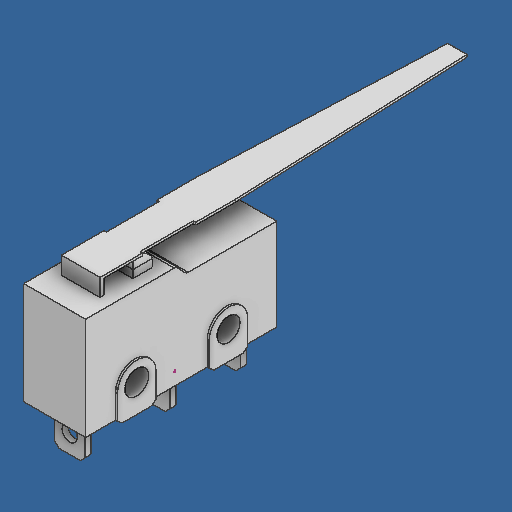
# Autodesk Inventor part: limit_switch
Saved by Autodesk Inventor 2026.2 (Build 302298000, 298)
## iProperties
Created: 2026-01-30
Part Number: limit_switch
Material: Generic
Document SubType Name: Modeling
Designer: Thoma
Density: 1 g/cm^3
Appearance: Default
Author: Thoma
Autodesk Inventor part; units mm, degrees
ref_plane "YZ Plane" through (0, 0, 0) normal (1, 0, 0) x (0, 1, 0)
ref_plane "XZ Plane" through (0, 0, 0) normal (0, 1, 0) x (-1, 0, 0)
ref_plane "XY Plane" through (0, 0, 0) normal (0, 0, 1) x (1, 0, 0)
sketch "Sketch4" plane through (0, 0, 0) normal (1, 0, 0) x (0, 1, 0)
  line L0 (9.275, 9.2) -> (-1.325, 9.2)
  line L1 (-1.325, 9.2) -> (-1.325, -10.6)
  line L2 (-1.325, -10.6) -> (9.275, -10.6)
  line L3 (9.275, -10.6) -> (9.275, 9.2)
  line L4 (-1.325, -0.7) -> (8.175, -0.7)
  line L5 (8.175, -0.7) -> (8.175, -10.6)
  line L6 (8.175, -10.6) -> (-1.325, -10.6)
  line L7 (-1.325, -10.6) -> (-1.325, -0.7)
  line L8 (9.275, -0.2) -> (8.175, -1.2)
  circle A0 centre (1.175, 4.1) radius 1.25
  line L9 (-1.725, 5.6) -> (-1.725, 2.6)
  line L10 (-1.725, 5.6) -> (-1.325, 6.1)
  line L11 (-1.725, 2.6) -> (-1.325, 2.1)
  line L12 (1.175, 4.1) -> (-1.325, 4.1)
  circle A1 centre (1.175, 4.1) radius 2
  line L13 (1.175, 6.1) -> (-1.325, 6.1)
  line L14 (1.175, 2.1) -> (-1.325, 2.1)
  circle A2 centre (1.175, -5.4) radius 1.2
  point P0 (0, 0)
  point P1 (9.275, -0.7)
  dimension "d11" = 10.6
  dimension "d12" = 9.5
  dimension "d13" = 0.5
  dimension "d14" = 0.5
  dimension "d15" = 19.8
  dimension "d16" = 2.5
  dimension "d17" = 2.5
  dimension "d18" = 5.1
  dimension "d19" = 0.4
  dimension "d20" = 2
  dimension "d21" = 2
  dimension "d22" = 0.5
  dimension "d23" = 0.5
  dimension "d24" = 4
  dimension "d37" = 9.5
  dimension "d38" = 2.4
  constraints: 30 end point, 6 point on line, 4 parallel, 3 centre point, 3 horizontal, 3 perpendicular, 2 coincident, 2 midpoint, 2 point on circle, 1 tangent, 1 vertical
  measures "d11" distance of L0.start L0.end
  measures "d12" distance of L4.start L4.end
  measures "d13" distance of L4.end L8.end
  measures "d14" distance of point (9.275, -0.7) L8.start
  measures "d15" distance of L0.end L1.end
  measures "d16" diameter of A0
  measures "d17" distance from line of L1 L12.start
  measures "d18" distance from line of L0 L12.start
  measures "d19" distance between parallel lines of L1 L9
  measures "d20" distance of L12.end L10.end
  measures "d21" distance of L11.end L12.end
  measures "d22" vertical distance of L10.end L9.start
  measures "d23" vertical distance of L11.end L9.end
  measures "d24" diameter of A1
  measures "d37" distance of point (1.175, -5.4) L12.start
  measures "d38" diameter of A2
extrude "Extrusion4" add sketch "Sketch4" against normal blind 6.4 contours L3 L8 L5 L4 L1 L14 A1 L13 L0 | L13 A1 L12 L1 | L1 L11 L9 L10 | L5 L2 L1 L4 | L12 A1 L14 L1 | A1
sketch "Sketch5" plane through (0, 0, 0) normal (1, 0, 0) x (0, 0, -1)
  line L0 (-6.1, -1.325) -> (-6.1, 1.102)
  line L1 (10.6, -1.325) -> (-2.1, -1.325) projected
  line L2 (-2.1, -1.325) -> (-2.1, 1.102)
  circle A0 centre (-4.1, 1.175) radius 1.25 projected
  arc A1 (-2.1, 1.175) -> (-6.1, 1.175) centre (-4.1, 1.175) ccw
  line L3 (-9.2, -1.325) -> (-6.1, -1.325) projected
  line L4 (-6.1, -1.325) -> (-5.6, -1.725) projected
  line L5 (-6.1, -1.325) -> (-5.6, -1.725)
  line L6 (-5.6, -1.725) -> (-2.6, -1.725) projected
  line L7 (-5.6, -1.725) -> (-2.6, -1.725)
  line L8 (-2.6, -1.725) -> (-2.1, -1.325)
  circle A2 centre (5.4, 1.175) radius 1.2
  arc A3 (7.4, 1.175) -> (3.4, 1.175) centre (5.4, 1.175) ccw
  line L9 (3.4, 1.175) -> (3.4, -1.325)
  line L10 (7.4, 1.175) -> (7.4, -1.325)
  line L11 (3.9, -1.725) -> (6.9, -1.725)
  line L12 (3.4, -1.325) -> (3.9, -1.725)
  line L13 (6.9, -1.725) -> (7.4, -1.325)
  line L14 (-6.1, 1.102) -> (-6.1, 1.175)
  line L15 (-2.1, 1.175) -> (-2.1, 1.102)
  point P0 (0, 0)
  dimension "d27" = 4
  dimension "d28" = 9.5
  dimension "d29" = 2.5
  dimension "d30" = 2.4
  dimension "d31" = 4
  dimension "d32" = 0.5
  dimension "d33" = 0.5
  dimension "d34" = 0.4
  constraints: 24 end point, 4 point on circle, 4 point on line, 4 vertical, 3 centre point, 3 coincident, 2 collinear, 2 perpendicular, 1 horizontal, 1 tangent
  measures "d27" diameter of A1
  measures "d28" distance of point (5.4, 1.175) A1.centre
  measures "d29" distance from line of L1 point (5.4, 1.175)
  measures "d30" diameter of A2
  measures "d31" diameter of A3
  measures "d32" horizontal distance of L9.end L11.start
  measures "d33" horizontal distance of L10.end L11.end
  measures "d34" distance between parallel lines of L11 L1
extrude "Extrusion5" add sketch "Sketch5" along normal blind 0.2
sketch "Sketch6" plane through (0, 0, 0) normal (1, 0, 0) x (0, 0, -1)
  point P0 (0, 0)
sketch "Sketch7" plane through (0, 0, 0) normal (-1, 0, 0) x (0, 0, 1)
  circle A0 centre (-5.4, 1.175) radius 1.2 projected
  line L0 (-3.9, -1.725) -> (-6.9, -1.725) projected
  line L1 (-5.4, 1.175) -> (-3.9, -1.725)
  line L2 (-3.4, -1.325) -> (-3.9, -1.725) projected
  line L3 (-3.9, -1.725) -> (-3.4, -1.325)
  line L4 (-7.4, -1.325) -> (-10.6, -1.325) projected
  line L5 (-3.4, -1.325) -> (-7.4, -1.325)
  line L6 (-7.4, -1.325) -> (-6.9, -1.725)
  line L7 (-6.9, -1.725) -> (-7.4, -1.325) projected
  point P0 (0, 0)
  constraints: 8 end point, 2 collinear, 1 point on line
extrude "Extrusion6" add sketch "Sketch7" along normal blind 6.4 contours L0 L6 L5 L1 | L1 L5 L2
fillet "Fillet1" radius 0.5 2 edges at (-3.2, 8.175, -1.2) (-3.2, 9.275, -0.2)
sketch "Sketch8" plane through (-6.4, 0, 0) normal (-1, 0, 0) x (0, 0, 1)
  circle A0 centre (-5.4, 1.175) radius 1.2 projected
  circle A1 centre (-5.4, 1.175) radius 1.2
  circle A2 centre (4.1, 1.175) radius 1.25 projected
  circle A3 centre (4.1, 1.175) radius 1.25
  circle A4 centre (-5.4, 1.175) radius 2
  circle A5 centre (4.1, 1.175) radius 2
  line L0 (-3.4, -1.325) -> (2.1, -1.325) projected
  line L1 (-3.4, -1.325) -> (-3.4, 1.175)
  line L2 (-10.6, -1.325) -> (-7.4, -1.325) projected
  line L3 (-7.4, 1.175) -> (-7.4, -1.325) projected
  line L4 (-7.4, -1.325) -> (-7.4, 1.175)
  line L5 (-7.4, -1.325) -> (-6.9, -1.725) projected
  line L6 (-7.4, -1.325) -> (-6.9, -1.725)
  line L7 (-6.9, -1.725) -> (-3.9, -1.725) projected
  line L8 (-6.9, -1.725) -> (-3.9, -1.725)
  line L9 (-3.9, -1.725) -> (-3.4, -1.325)
  line L10 (2.1, -1.325) -> (2.1, 1.175)
  line L11 (6.1, -1.325) -> (9.2, -1.325) projected
  line L12 (6.1, -1.325) -> (6.1, 1.175)
  line L13 (2.6, -1.725) -> (2.1, -1.325) projected
  line L14 (2.1, -1.325) -> (2.6, -1.725)
  line L15 (2.6, -1.725) -> (5.6007, -1.725)
  line L16 (5.6007, -1.725) -> (6.1, -1.325)
  point P0 (0, 0)
  dimension "d42" = 2.5
  dimension "d43" = 4
  dimension "d44" = 4
  constraints: 20 end point, 4 centre point, 4 coincident, 4 collinear, 3 point on circle, 3 tangent, 1 perpendicular
  measures "d42" diameter of A3
  measures "d43" diameter of A4
  measures "d44" diameter of A5
extrude "Extrusion7" add sketch "Sketch8" along normal blind 0.2
sketch "Sketch10" plane through (-6.4, 9.275, 9.2) normal (0, 1, 0) x (1, 0, 0)
  line L0 (6.6, 12.6) -> (6.6, 16.6) projected
  line L1 (6.6, 14.6) -> (3.2, 14.6)
  line L2 (3.2, 14.6) -> (3.2, 7.1)
  line L3 (1.2, 8.1) -> (5.2, 8.1)
  line L4 (5.2, 8.1) -> (5.2, 6.1)
  line L5 (5.2, 6.1) -> (1.2, 6.1)
  line L6 (1.2, 6.1) -> (1.2, 8.1)
  point P0 (6.4, 9.2)
  dimension "d48" = 3.4
  dimension "d49" = 7.5
  dimension "d50" = 1
  dimension "d51" = 2
  dimension "d52" = 4
  dimension "d53" = 2
  constraints: 12 end point, 2 horizontal, 2 parallel, 1 midpoint, 1 perpendicular, 1 vertical
  measures "d48" distance of L1.start L1.end
  measures "d49" distance of L1.end L2.end
  measures "d50" distance from line of L5 L2.end
  measures "d51" distance from line of L2.end L6
  measures "d52" distance of L4.end L5.end
  measures "d53" distance of L3.end L4.end
extrude "Extrusion8" add sketch "Sketch10" along normal blind 1.3
sketch "Sketch11" plane through (-6.4, 9.275, 9.2) normal (0, 1, 0) x (1, 0, 0)
  line L0 (1.2, 6.1) -> (5.2, 6.1) projected
  line L1 (3.2, 6.1) -> (3.2, 3.1)
  line L2 (3.2, 3.1) -> (5.2, 3.1)
  line L3 (6.4, 3.1) -> (0, 3.1) projected
  line L4 (5.2, 2.7) -> (1.2, 2.7)
  line L5 (1.2, 2.7) -> (1.2, 3.1)
  line L6 (-0.2, 3.85) -> (6.6, 3.85) projected
  line L7 (3.2, 3.1) -> (1.2, 3.1)
  line L8 (5.2, 2.7) -> (5.2, 3.1)
  point P0 (6.4, 9.2)
  point P1 (3.2, 3.1)
  dimension "d56" = 3
  dimension "d57" = 0.4
  dimension "d58" = 4
  dimension "d59" = 2
  constraints: 12 end point, 2 midpoint, 2 point on line, 2 vertical, 1 horizontal, 1 perpendicular
  measures "d56" distance of L1.start L1.end
  measures "d57" distance of L4.start L2.end
  measures "d58" distance of L4.start L4.end
  measures "d59" distance from line of L8 point (3.2, 3.1)
extrude "Extrusion9" add sketch "Sketch11" along normal blind 1.8
sketch "Sketch12" plane through (-1.2, 9.275, 6.1) normal (0, 0, -1) x (-1, 0, 0)
  line L0 (4, 1.3) -> (0, 1.3) projected
  line L1 (0, 1.8) -> (4, 1.8)
  line L2 (4, 1.8) -> (4, 1.3)
  line L3 (4, 1.3) -> (0, 1.3)
  line L4 (0, 1.3) -> (0, 1.8)
  line L5 (0, 1.8) -> (4, 1.8)
  line L6 (4, 1.8) -> (4, 1.55)
  line L7 (4, 1.55) -> (0, 1.55)
  line L8 (0, 1.55) -> (0, 1.8)
  point P0 (-1.2, -9.275)
  point P1 (0, 1.3)
  point P2 (0, 1.55)
  constraints: 16 end point, 4 parallel, 2 horizontal, 2 perpendicular, 1 midpoint
extrude "Extrusion10" add sketch "Sketch12" along normal blind 38.6 contours L7 L4 L1 L2
sketch "Sketch13" plane through (0, -1.325, -3.4) normal (0, -1, 0) x (1, 0, 0)
  line L0 (0, 12.6) -> (-6.4, 12.6) projected
  line L1 (-3.2, 12.6) -> (-3.2, -7.2)
  line L2 (0, -7.2) -> (-6.4, -7.2) projected
  line L3 (-1.6, 2.25) -> (-4.8, 2.25)
  line L4 (-4.8, 2.25) -> (-4.8, 1.65)
  line L5 (-4.8, 1.65) -> (-1.6, 1.65)
  line L6 (-1.6, 1.65) -> (-1.6, 2.25)
  line L7 (-1.6, -5.05) -> (-4.8, -5.05)
  line L8 (-4.8, -5.05) -> (-4.8, -5.65)
  line L9 (-4.8, -5.65) -> (-1.6, -5.65)
  line L10 (-1.6, -5.65) -> (-1.6, -5.05)
  line L11 (-1.6, 11.05) -> (-4.8, 11.05)
  line L12 (-4.8, 11.05) -> (-4.8, 10.45)
  line L13 (-4.8, 10.45) -> (-1.6, 10.45)
  line L14 (-1.6, 10.45) -> (-1.6, 11.05)
  point P0 (0, 3.4)
  point P1 (-3.2, 10.75)
  point P2 (-3.2, 1.95)
  point P3 (-3.2, -5.35)
  dimension "d64" = 1.85
  dimension "d65" = 8.8
  dimension "d66" = 7.3
  dimension "d67" = 3.2
  dimension "d68" = 0.6
  dimension "d69" = 0.3
  dimension "d70" = 1.6
  dimension "d71" = 3.2
  dimension "d72" = 0.6
  dimension "d73" = 0.3
  dimension "d74" = 1.6
  dimension "d75" = 3.2
  dimension "d76" = 0.6
  dimension "d77" = 1.6
  dimension "d78" = 0.3
  constraints: 26 end point, 6 parallel, 3 horizontal, 3 perpendicular, 3 point on line, 2 midpoint
  measures "d64" distance from line of L0 point (-3.2, 10.75)
  measures "d65" distance of point (-3.2, 1.95) point (-3.2, 10.75)
  measures "d66" distance of point (-3.2, -5.35) point (-3.2, 1.95)
  measures "d67" distance of L4.end L5.end
  measures "d68" distance of L5.end L3.start
  measures "d69" distance from line of point (-3.2, 1.95) L5
  measures "d70" distance from line of point (-3.2, 1.95) L6
  measures "d71" distance of L8.end L9.end
  measures "d72" distance of L9.end L7.start
  measures "d73" distance from line of point (-3.2, -5.35) L9
  measures "d74" distance from line of point (-3.2, -5.35) L10
  measures "d75" distance of L12.end L13.end
  measures "d76" distance of L13.end L11.start
  measures "d77" distance from line of point (-3.2, 10.75) L14
  measures "d78" distance from line of point (-3.2, 10.75) L13
extrude "Extrusion11" add sketch "Sketch13" along normal blind 3.9
chamfer "Chamfer1" distance 0.5 angle 45 6 edges at (-1.6, -5.225, 7.35) (-4.8, -5.225, 7.35) (-4.8, -5.225, -1.45) (-1.6, -5.225, -1.45) (-1.6, -5.225, -8.75) (-4.8, -5.225, -8.75)
sketch "Sketch14" plane through (-4.8, -1.325, 7.65) normal (0, 0, 1) x (1, 0, 0)
  circle A0 centre (1.6, -2) radius 0.8
  point P0 (4.8, 1.325)
  dimension "d84" = 1.6
  constraints: 1 centre point
  measures "d84" diameter of A0
extrude "Extrusion12" cut sketch "Sketch14" against normal blind 19
chamfer "Chamfer2" distance 1 distance2 25 2 edges at (-5.2, 10.95, -32.5) (-1.2, 10.95, -32.5) measured on face at (-2.5333, 10.9917, -32.5)
sketch "Sketch15" plane through (-6.4, 11.075, 9.2) normal (0, 1, 0) x (1, 0, 0)
  line L0 (6.4, 7.1) -> (0, 7.1) projected
  line L1 (0, 12.6) -> (6.4, 12.6) projected
  line L2 (1.2, 7.1) -> (1.45, 7.1)
  line L3 (1.45, 7.1) -> (1.45, 12.6)
  line L4 (1.45, 12.6) -> (1.2, 12.6)
  line L5 (1.2, 12.6) -> (1.2, 7.1)
  line L6 (5.2, 7.1) -> (4.95, 7.1)
  line L7 (4.95, 7.1) -> (4.95, 12.6)
  line L8 (4.95, 12.6) -> (5.2, 12.6)
  line L9 (5.2, 12.6) -> (5.2, 7.1)
  line L10 (5.2, 2.7) -> (5.2, 16.7) projected
  line L11 (1.2, 2.7) -> (1.2, 16.7) projected
  point P0 (6.4, 9.2)
  point P1 (1.2, 12.6)
  point P2 (1.45, 7.1)
  dimension "d90" = 0.25
  dimension "d91" = 0
  dimension "d92" = 0
  dimension "d93" = 0.25
  constraints: 16 end point, 4 parallel, 4 point on line, 2 horizontal, 2 perpendicular
  measures "d90" distance between parallel lines of L7 L9
  measures "d91" distance between parallel lines of L10 L9
  measures "d92" distance between parallel lines of L11 L5
  measures "d93" distance between parallel lines of L5 L3
extrude "Extrusion13" cut sketch "Sketch15" against normal blind 0.4 contours L0 L7 L1 L9 | L0 L5 L1 L3
fillet "Fillet2" radius 0.5 4 edges at (-3.2, 10.575, 1.1) (-1.2, 10.575, 2.1) (-5.2, 10.575, 2.1) (-3.2, 10.575, 3.1)
body "Solid2"
